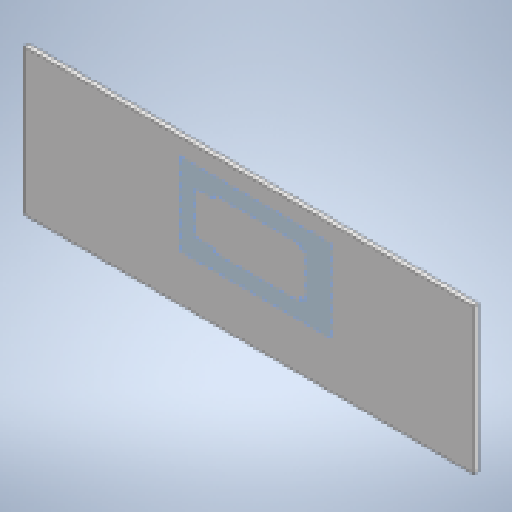
# Autodesk Inventor part: backplate
Saved by Autodesk Inventor 2023 (Build 270158030, 158C)
## iProperties
Created: 2024-09-24
Part Number: backplate
Material: Generic
Document SubType Name: Modeling
Designer: Imogen Heard
Density: 1 g/cm^3
Appearance: Default
Author: Imogen Heard
Autodesk Inventor part; units mm, degrees
ref_plane "YZ Plane" through (0, 0, 0) normal (1, 0, 0) x (0, 1, 0)
ref_plane "XZ Plane" through (0, 0, 0) normal (0, 1, 0) x (-1, 0, 0)
ref_plane "XY Plane" through (0, 0, 0) normal (0, 0, 1) x (1, 0, 0)
sketch "Sketch1" plane through (0, 0, 0) normal (0, 0, 1) x (1, 0, 0)
  line L0 (90.331, -15) -> (-48.669, -15)
  line L1 (-48.669, -15) -> (-48.669, 30)
  line L2 (-48.669, 30) -> (90.331, 30)
  line L3 (90.331, 30) -> (90.331, -15)
  line L4 (3.6008, 15) -> (3.6008, 14) projected
  line L5 (3.6008, 15) -> (38.0611, 15) projected
  line L6 (38.0611, 15) -> (38.0611, 14) projected
  line L7 (38.0611, 14) -> (3.6008, 14) projected
  arc A0 (1.6411, 15) -> (0, 14) centre (6, 6) ccw projected
  line L8 (0, 14) -> (34.0626, 14) projected
  line L9 (34.0626, 15) -> (34.0626, 14) projected
  line L10 (34.0626, 15) -> (1.6411, 15) projected
  line L11 (3.6008, 15) -> (-2.0587, 15) projected
  line L12 (-17.3084, 15) -> (-2.0587, 15) projected
  line L13 (38.0611, 0) -> (3.6008, 0) projected
  line L14 (-2.0587, 0) -> (3.6008, 0) projected
  line L15 (70.331, 14) -> (63.6008, 14) projected
  arc A1 (70.331, 1) -> (70.331, 14) centre (70.331, 7.5) ccw projected
  line L16 (63.6008, 1) -> (70.331, 1) projected
  line L17 (63.6008, 14) -> (63.6008, 1) projected
  line L18 (-21.9389, 14) -> (-28.669, 14) projected
  line L19 (-21.9389, 1) -> (-21.9389, 14) projected
  line L20 (-28.669, 1) -> (-21.9389, 1) projected
  arc A2 (-28.669, 14) -> (-28.669, 1) centre (-28.669, 7.5) ccw projected
  arc A3 (-28.669, 15) -> (-28.669, 0) centre (-28.669, 7.5) ccw projected
  arc A4 (70.331, 0) -> (70.331, 15) centre (70.331, 7.5) ccw projected
  point P0 (0, 0)
  point P1 (20.831, 30)
  dimension "d0" = 15
  dimension "d1" = 15
  dimension "d2" = 20
  dimension "d3" = 20
  constraints: 8 end point, 2 parallel, 1 horizontal, 1 midpoint, 1 perpendicular
  measures "d0" distance from line of L0 point (0, 0)
  measures "d1" distance from line of L5 point (20.831, 30)
  measures "d2" distance from line of L3 A1.centre
  measures "d3" distance from line of L1 A2.centre
extrude "Extrusion1" add sketch "Sketch1" along normal blind 1.5 contours L0 L1 L2 L3 | L5 L9 L7 L4 | L4 L8 A0 L10 | L5 L6 L7 L9 | A1 L16 L17 L15 | L19 L20 A2 L18
sketch "Sketch2" plane through (0, 0, 0) normal (0, 0, -1) x (-1, 0, 0)
  line L0 (-6, 15) -> (-6, 0) projected
  line L1 (-31.6619, 15) -> (-6, 15) projected
  line L2 (-31.6619, 0) -> (-31.6619, 15) projected
  line L3 (-31.6619, 0) -> (-6, 0) projected
  line L4 (-90.331, 30) -> (48.669, 30) projected
  line L5 (-90.331, 30) -> (48.669, 30) projected
  line L6 (-90.331, -15) -> (-90.331, 30) projected
  line L7 (48.669, -15) -> (-90.331, -15) projected
  line L8 (48.669, 30) -> (48.669, -15) projected
  line L9 (-5.8, 15.2) -> (-5.8, -0.2)
  line L10 (-5.8, -0.2) -> (-31.8619, -0.2)
  line L11 (-31.8619, -0.2) -> (-31.8619, 15.2)
  line L12 (-31.8619, 15.2) -> (-5.8, 15.2)
  line L13 (-41.8619, 20.2) -> (5, 20.2)
  line L14 (5, 20.2) -> (5, -5.2)
  line L15 (5, -5.2) -> (-41.8619, -5.2)
  line L16 (-41.8619, -5.2) -> (-41.8619, 20.2)
  line L17 (-34.0626, 1) -> (0, 1) projected
  line L18 (-34.0626, 14) -> (-34.0626, 1) projected
  line L19 (0, 14) -> (-34.0626, 14) projected
  line L20 (0, 1) -> (0, 14) projected
  point P0 (0, 0)
  point P1 (-31.8619, 1)
  point P2 (-31.8619, 14)
  point P3 (-5.8, 14)
  point P4 (-5.8, 1)
  dimension "d6" = 0.2
  dimension "d7" = 5
  dimension "d8" = 10
  dimension "d9" = 5
  dimension "d10" = 5
  constraints: 16 end point, 2 parallel, 1 horizontal, 1 perpendicular, 3 other
  measures "d6" distance between parallel lines of L12 L1
  measures "d7" distance between parallel lines of L13 L12
  measures "d8" distance between parallel lines of L11 L16
  measures "d9" distance between parallel lines of L15 L10
  measures "d10" distance between parallel lines of L14 L20
extrude "Extrusion2" add sketch "Sketch2" along normal blind 3 contours L13 L14 L15 L16
body "Solid1"
